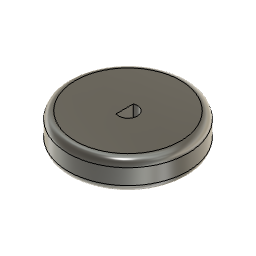
Full-Cat v5 (Autodesk Fusion 360 archive; units mm, degrees)
design "wheel v2"
Autodesk Fusion 360 part; units mm, degrees
sketch "Sketch1" plane through (0, 0, 0) normal (0, 0, 1) x (1, 0, 0)
  circle A0 centre (0, 0) radius 10
  dimension "d1" = 20
  constraint coincident A0.centre origin
  measures "d1" diameter of A0
extrude "Extrude1" add sketch "Sketch1" along normal blind 5
fillet "Fillet1" radius 1.2 2 edges at (-9.3233, -3.6162, 5) (-9.3233, -3.6162, 0)
sketch "Sketch2" plane through (0, 0, 5) normal (0, 0, 1) x (-1, 0, 0)
  circle A0 centre (0, 0) radius 8.8
  circle A1 centre (0, 0) radius 1.55
  line L0 (0.55, 1.4491) -> (2.3002, 1.4491)
  line L1 (2.3002, 1.4491) -> (2.3002, -1.4465)
  line L2 (2.3002, -1.4465) -> (0.55, -1.4465)
  line L3 (0.55, -1.4465) -> (0.55, 1.4491)
  dimension "d6" = 3.1
  dimension "d7" = 0.55
  constraint concentric A0 A1
  constraint horizontal L0
  constraint vertical L1
  constraint horizontal L2
  constraint vertical L3
  constraint coincident A1 L0.start
  measures "d6" diameter of A1
  measures "d7" distance of A0.centre L3
extrude "Extrude2" cut sketch "Sketch2" against normal blind 50 contours A1 L2 L3 picked at (-0.1284, 0.5)

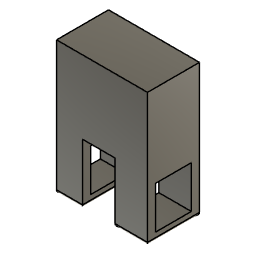
design "leg v11"
Autodesk Fusion 360 part; units mm, degrees
sketch "Sketch1" plane through (0, 0, 0) normal (0, 0, 1) x (1, 0, 0)
  line L0 (0, 0) -> (60, 0)
  line L1 (60, 0) -> (60, 20)
  line L2 (60, 20) -> (0, 20)
  line L3 (0, 20) -> (0, 0)
  dimension "d1" = 60
  dimension "d2" = 20
  constraint horizontal L0
  constraint vertical L1
  constraint horizontal L2
  constraint vertical L3
  constraint coincident L0.start L3.end
  measures "d1" distance of L0.start L0.end
  measures "d2" distance of L0.start L2.end
extrude "Extrude1" add sketch "Sketch1" along normal blind 40
sketch "Sketch2" plane through (0, 0, 0) normal (-1, 0, 0) x (0, -1, 0)
  line L0 (-20, 0) -> (0, 0)
  line L1 (0, 0) -> (0, 40)
  line L2 (0, 40) -> (-20, 40)
  line L3 (-20, 40) -> (-20, 0)
  line L4 (-15, 28) -> (-5, 28)
  line L5 (-5, 28) -> (-5, 16)
  line L6 (-5, 16) -> (-15, 16)
  line L7 (-15, 16) -> (-15, 28)
  dimension "d5" = 10
  dimension "d6" = 12
  dimension "d7" = 5
  constraint horizontal L4
  constraint vertical L5
  constraint horizontal L6
  constraint vertical L7
  measures "d5" distance of L4.start L4.end
  measures "d6" distance of L4.start L6.end
  measures "d7" distance of L3 L7
extrude "Extrude2" cut sketch "Sketch2" against normal blind 30 contours L4 L5 L6 L7
extrude "Extrude3" cut 1 faces at (20, 13.3333, 40) along direction (0, 0, -1) blind 2
extrude "Extrude4" cut 1 faces at (20, 13.3333, 0) along direction (0, 0, 1) blind 2
sketch "Sketch3" plane through (0, 20, 0) normal (0, 1, 0) x (-1, 0, 0)
  line L0 (-60, 2) -> (0, 2)
  line L1 (0, 2) -> (0, 38)
  line L2 (0, 38) -> (-60, 38)
  line L3 (-60, 38) -> (-60, 2)
  line L4 (-40, 33) -> (-20, 33)
  line L5 (-20, 33) -> (-20, -1)
  line L6 (-20, -1) -> (-40, -1)
  line L7 (-40, -1) -> (-40, 33)
  dimension "d14" = 20
  dimension "d15" = 34
  dimension "d16" = 20
  dimension "d17" = 5
  constraint horizontal L4
  constraint vertical L5
  constraint horizontal L6
  constraint vertical L7
  measures "d14" distance of L4.start L4.end
  measures "d15" distance of L4.start L6.end
  measures "d16" distance of L3 L7
  measures "d17" distance of L2 L4
extrude "Extrude5" cut 1 faces at (20, 13.3333, 2) along direction (0, 0, 1) blind 9
extrude "Extrude6" cut 1 faces at (20, 13.3333, 11) along direction (0, 0, 1) blind 1
extrude "Extrude7" cut sketch "Sketch3" against normal blind 20 contours L0 L4 L5 L7
extrude "Extrude8" cut sketch "Sketch2" against normal blind 80 contours L4 L5 L6 L7
extrude "Extrude9" cut 1 faces at (20, 13.3333, 38) along direction (0, 0, -1) blind 1
extrude "Extrude10" cut 1 faces at (60, 8.3333, 34) along direction (-1, 0, 0) blind 10
extrude "Extrude11" add 1 faces at (40, 1.6667, 24.3333) along direction (-1, 0, 0) blind 10
extrude "Extrude12" cut 1 faces at (50, 8.3333, 34) along direction (-1, 0, 0) blind 10
extrude "Extrude13" cut 1 faces at (6.6667, 20, 27.3333) along direction (0, -1, 0) blind 2
extrude "Extrude14" cut 1 faces at (6.6667, 0, 27.3333) along direction (0, 1, 0) blind 2
extrude "Extrude15" cut 1 faces at (36.6667, 12.6667, 12) along direction (0, 0, 1) blind 1
extrude "Extrude16" cut 1 faces at (13.3333, 7.3333, 12) along direction (0, 0, 1) blind 1
extrude "Extrude17" cut 1 faces at (36.6667, 12.6667, 13) along direction (0, 0, 1) blind 1
extrude "Extrude18" cut 1 faces at (13.3333, 7.3333, 13) along direction (0, 0, 1) blind 1
extrude "Extrude19" cut sketch "Sketch2" against normal blind 2
extrude "Extrude20" cut 1 faces at (14.6667, 7.3333, 37) along direction (0, 0, -1) blind 1
extrude "Extrude21" add 1 faces at (26.6667, 12.6667, 33) along direction (0, 0, -1) blind 1
extrude "Extrude22" cut 1 faces at (14.6667, 7.3333, 36) along direction (0, 0, -1) blind 1
fillet "Fillet1" radius 1 2 faces at (36.6667, 12.6667, 14) (14, 7.3333, 14)
sketch "Sketch4" plane through (2, 0, 0) normal (-1, 0, 0) x (0, -1, 0)
  line L0 (-5, 16) -> (-15, 16)
  line L1 (-15, 16) -> (-15, 28)
  line L2 (-15, 28) -> (-5, 28)
  line L3 (-5, 28) -> (-5, 16)
  line L4 (-18, 15) -> (-2, 15)
  line L5 (-2, 15) -> (-2, 35)
  line L6 (-2, 35) -> (-18, 35)
  line L7 (-18, 35) -> (-18, 15)
  line L8 (-15.5, 28.5) -> (-4.5, 28.5)
  line L9 (-4.5, 28.5) -> (-4.5, 15.5)
  line L10 (-4.5, 15.5) -> (-15.5, 15.5)
  line L11 (-15.5, 15.5) -> (-15.5, 28.5)
  dimension "d56" = 11
  dimension "d57" = 13
  dimension "d58" = 2.5
  dimension "d59" = 6.5
  constraint horizontal L8
  constraint vertical L9
  constraint horizontal L10
  constraint vertical L11
  measures "d56" distance of L8.start L8.end
  measures "d57" distance of L8.start L10.end
  measures "d58" distance of L7 L11
  measures "d59" distance of L6 L8
extrude "Extrude23" cut sketch "Sketch4" against normal blind 50 contours L8 L9 L10 L11
extrude "Extrude24" add 2 faces at (36.6667, 8.1667, 15.5) (14, 11.8333, 15.5) along direction (0, 0, 1) blind 1
extrude "Extrude25" cut 2 faces at (33.3333, 11.8333, 28.5) (14, 11.8333, 28.5) along direction (0, 0, 1) blind 1
extrude "Extrude26" cut 1 faces at (26.6667, 12.6667, 32) along direction (0, 0, 1) blind 0.5
extrude "Extrude27" add 1 faces at (14.6667, 7.3333, 35) along direction (0, 0, 1) blind 20
extrude "Extrude28" cut 1 faces at (2, 8.1667, 46.5) along direction (1, 0, 0) blind 10
extrude "Extrude29" cut 1 faces at (5.3333, 12.6667, 15) along direction (0, 0, -1) blind 15

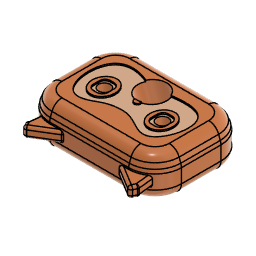
design "head v3"
Autodesk Fusion 360 part; units mm, degrees
sketch "Sketch1" plane through (0, 0, 0) normal (0, 0, 1) x (1, 0, 0)
  line L0 (10, 0) -> (40, 0)
  line L1 (50, 10) -> (50, 25)
  line L2 (40, 35) -> (10, 35)
  line L3 (0, 25) -> (0, 10)
  arc A0 (0, 10) -> (10, 0) centre (10, 10) ccw
  arc A1 (40, 0) -> (50, 10) centre (40, 10) ccw
  arc A2 (50, 25) -> (40, 35) centre (40, 25) ccw
  arc A3 (10, 35) -> (0, 25) centre (10, 25) ccw
  point P0 (50, 0)
  point P1 (0, 35)
  dimension "d1" = 50
  dimension "d2" = 35
  dimension "d3" = 10
  dimension "d4" = 10
  dimension "d5" = 10
  dimension "d6" = 10
  constraint horizontal L0
  constraint vertical L1
  constraint horizontal L2
  constraint vertical L3
  constraint coincident origin L0
  constraint coincident origin L3
  constraint tangent L0 A0
  constraint tangent L3 A0
  constraint coincident P0 L0
  constraint coincident P0 L1
  constraint tangent L0 A1
  constraint tangent L1 A1
  constraint tangent L1 A2
  constraint tangent L2 A2
  constraint coincident P1 L2
  constraint coincident P1 L3
  constraint tangent L2 A3
  constraint tangent L3 A3
  measures "d1" distance of origin P0
  measures "d2" distance of origin P1
  measures "d3" radius of A0
  measures "d4" radius of A1
  measures "d5" radius of A2
  measures "d6" radius of A3
extrude "Extrude1" add sketch "Sketch1" along normal blind 10 makes body 1
extrude "Extrude2" add 1 faces at (20, 23.3333, 10) along direction (0, 0, 1) blind 5 draft -20 on bodies 1 bodies 1
fillet "Fillet1" radius 4 16 faces at (9.2077, 34.0555, 12.5) (30, 34.3934, 11.6667) (49.0555, 25.7923, 12.5) (49.3934, 15, 11.6667) (49.0555, 9.2077, 12.5) (20, 0.6066, 11.6667) (9.2077, 0.9445, 12.5) (1.2132, 15, 13.3333) (0.2819, 27.3576, 6.6667) (0, 20, 3.3333) (8.1075, 0.1807, 6.6667) (20, 0, 3.3333) (40.4758, 0.0113, 6.6667) (50, 15, 3.3333) (40.4758, 34.9887, 6.6667) (30, 35, 3.3333) on bodies 1
sketch "Sketch2" plane through (0, 0, 15) normal (0, 0, 1) x (-1, 0, 0)
  arc A0 (-10, -30.3793) -> (-4.6207, -25) centre (-10, -25) ccw
  line L0 (-4.6207, -25) -> (-4.6207, -10)
  arc A1 (-4.6207, -10) -> (-10, -4.6207) centre (-10, -10) ccw
  line L1 (-10, -4.6207) -> (-40, -4.6207)
  arc A2 (-40, -4.6207) -> (-45.3793, -10) centre (-40, -10) ccw
  line L2 (-45.3793, -10) -> (-45.3793, -25)
  arc A3 (-45.3793, -25) -> (-40, -30.3793) centre (-40, -25) ccw
  line L3 (-40, -30.3793) -> (-10, -30.3793)
  spline S0 degree 5 poles (-30, -11) (-30.1783, -10.9228) (-30.547, -10.7574) (-31.1363, -10.4766) (-31.9947, -10.0363) (-33.1875, -9.3975) (-34.4939, -8.7332) (-35.9004, -8.1781) (-37.3826, -7.9333) (-38.9002, -8.1993) (-40.3935, -9.1277) (-41.777, -10.756) (-42.9392, -12.974) (-43.7599, -15.5782) (-44.125, -18.3111) (-43.9424, -20.9044) (-43.1572, -23.1215) (-41.7684, -24.7994) (-39.846, -25.8922) (-37.5109, -26.4441) (-34.9163, -26.5618) (-32.2287, -26.3888) (-29.6089, -26.0789) (-27.1947, -25.7719) (-25.0786, -25.5642) (-23.3123, -25.5105) (-22.1979, -25.6122) (-21.5328, -25.7732) (-21.165, -25.9181) (-21, -26) knots 0 0 0 0 0 0 0.04 0.08 0.12 0.16 0.2 0.24 0.28 0.32 0.36 0.4 0.44 0.48 0.52 0.56 0.6 0.64 0.68 0.72 0.76 0.8 0.84 0.88 0.92 0.96 1 1 1 1 1 1
  spline S1 degree 5 poles (-30, -11) (-29.7784, -11.1039) (-29.3296, -11.2982) (-28.6391, -11.549) (-27.6842, -11.8023) (-26.437, -11.984) (-25.1478, -12.0335) (-23.84, -11.9573) (-22.5543, -11.7675) (-21.3346, -11.4794) (-20.2112, -11.1086) (-19.1868, -10.6682) (-18.2159, -10.1651) (-17.224, -9.6104) (-16.1378, -9.036) (-14.9108, -8.5076) (-13.5535, -8.1426) (-12.1194, -8.0819) (-10.6872, -8.4572) (-9.346, -9.3624) (-8.176, -10.8165) (-7.2413, -12.7559) (-6.5937, -15.0609) (-6.2733, -17.5726) (-6.3103, -20.1129) (-6.7267, -22.5039) (-7.5371, -24.5856) (-8.75, -26.2385) (-10.3695, -27.3818) (-12.3961, -27.9646) (-14.8283, -27.9594) (-17.0966, -27.4759) (-18.9783, -26.8429) (-20.3128, -26.301) (-21, -26) knots 0 0 0 0 0 0 0.033333 0.066667 0.1 0.133333 0.166667 0.2 0.233333 0.266667 0.3 0.333333 0.366667 0.4 0.433333 0.466667 0.5 0.533333 0.566667 0.6 0.633333 0.666667 0.7 0.733333 0.766667 0.8 0.833333 0.866667 0.9 0.933333 0.966667 1 1 1 1 1 1
  point P0 (-34, -9)
  point P1 (-40, -9)
  point P2 (-43, -23)
  point P3 (-29, -26)
  point P4 (-25, -12)
  point P5 (-20, -11)
  point P6 (-16, -9)
  point P7 (-10, -9)
  point P8 (-7, -23)
extrude "Extrude3" cut sketch "Sketch2" against normal blind 0.5 contours S0 S1 bodies 1
sketch "Sketch3" plane through (0, 0, 14.5) normal (0, 0, 1) x (-1, 0, 0)
  spline S0 degree 5 poles (-21, -26) (-21.165, -25.9181) (-21.5328, -25.7732) (-22.1979, -25.6122) (-23.3123, -25.5105) (-25.0786, -25.5642) (-27.1947, -25.7719) (-29.6089, -26.0789) (-32.2287, -26.3888) (-34.9163, -26.5618) (-37.5109, -26.4441) (-39.846, -25.8922) (-41.7684, -24.7994) (-43.1572, -23.1215) (-43.9424, -20.9044) (-44.125, -18.3111) (-43.7599, -15.5782) (-42.9392, -12.974) (-41.777, -10.756) (-40.3935, -9.1277) (-38.9002, -8.1993) (-37.3826, -7.9333) (-35.9004, -8.1781) (-34.4939, -8.7332) (-33.1875, -9.3975) (-31.9947, -10.0363) (-31.1363, -10.4766) (-30.547, -10.7574) (-30.1783, -10.9228) (-30, -11) knots -1 -1 -1 -1 -1 -1 -0.96 -0.92 -0.88 -0.84 -0.8 -0.76 -0.72 -0.68 -0.64 -0.6 -0.56 -0.52 -0.48 -0.44 -0.4 -0.36 -0.32 -0.28 -0.24 -0.2 -0.16 -0.12 -0.08 -0.04 0 0 0 0 0 0
  spline S1 degree 5 poles (-30, -11) (-29.7784, -11.1039) (-29.3296, -11.2982) (-28.6391, -11.549) (-27.6842, -11.8023) (-26.437, -11.984) (-25.1478, -12.0335) (-23.84, -11.9573) (-22.5543, -11.7675) (-21.3346, -11.4794) (-20.2112, -11.1086) (-19.1868, -10.6682) (-18.2159, -10.1651) (-17.224, -9.6104) (-16.1378, -9.036) (-14.9108, -8.5076) (-13.5535, -8.1426) (-12.1194, -8.0819) (-10.6872, -8.4572) (-9.346, -9.3624) (-8.176, -10.8165) (-7.2413, -12.7559) (-6.5937, -15.0609) (-6.2733, -17.5726) (-6.3103, -20.1129) (-6.7267, -22.5039) (-7.5371, -24.5856) (-8.75, -26.2385) (-10.3695, -27.3818) (-12.3961, -27.9646) (-14.8283, -27.9594) (-17.0966, -27.4759) (-18.9783, -26.8429) (-20.3128, -26.301) (-21, -26) knots 0 0 0 0 0 0 0.033333 0.066667 0.1 0.133333 0.166667 0.2 0.233333 0.266667 0.3 0.333333 0.366667 0.4 0.433333 0.466667 0.5 0.533333 0.566667 0.6 0.633333 0.666667 0.7 0.733333 0.766667 0.8 0.833333 0.866667 0.9 0.933333 0.966667 1 1 1 1 1 1
  ellipse E0 centre (-37.25, -19.25) end of major axis (-37.25, -14.25) minor radius 4.35
  line L0 (-37.25, -24.25) -> (-37.25, -14.25) construction
  line L1 (-32.9, -19.25) -> (-41.6, -19.25) construction
  ellipse E1 centre (-14, -18) end of major axis (-14, -13) minor radius 4.3564
  line L2 (-14, -23) -> (-14, -13) construction
  line L3 (-9.6436, -18) -> (-18.3564, -18) construction
  line L4 (-38, -16) -> (-36.5, -16)
  line L5 (-34.5, -18) -> (-34.5, -20.5)
  line L6 (-36.5, -22.5) -> (-38, -22.5)
  line L7 (-40, -20.5) -> (-40, -18)
  arc A0 (-38, -16) -> (-40, -18) centre (-38, -18) ccw
  arc A1 (-34.5, -18) -> (-36.5, -16) centre (-36.5, -18) ccw
  arc A2 (-36.5, -22.5) -> (-34.5, -20.5) centre (-36.5, -20.5) ccw
  arc A3 (-40, -20.5) -> (-38, -22.5) centre (-38, -20.5) ccw
  point P0 (-40, -16)
  point P1 (-40, -22.5)
  dimension "d15" = 5.5
  dimension "d16" = 6.5
  dimension "d17" = 2
  dimension "d18" = 8.7
  dimension "d19" = 1.6
  dimension "d20" = 1.75
  constraint coincident E0 L0.start
  constraint coincident E0 L0.end
  constraint coincident E0 L1.start
  constraint coincident E0 L1.end
  constraint vertical L0
  constraint coincident E1 L2.start
  constraint coincident E1 L2.end
  constraint coincident E1 L3.start
  constraint coincident E1 L3.end
  constraint vertical L2
  constraint horizontal L4
  constraint vertical L5
  constraint horizontal L6
  constraint vertical L7
  constraint coincident P0 L4
  constraint coincident P0 L7
  constraint tangent L4 A0
  constraint tangent L7 A0
  constraint tangent L4 A1
  constraint tangent L5 A1
  constraint equal A0 A1
  constraint tangent L5 A2
  constraint tangent L6 A2
  constraint equal A0 A2
  constraint coincident P1 L6
  constraint coincident P1 L7
  constraint tangent L6 A3
  constraint tangent L7 A3
  constraint equal A0 A3
  measures "d16" distance of P0 P1
  measures "d17" radius of A0
  measures "d19" distance of L1.end L7
  measures "d20" distance of L0.end L4
extrude "Extrude4" add sketch "Sketch3" along normal blind 0.5 separate body contours E0 makes body 2
move_body "Move1" bodies 2 to x (1, 0, 0) y (0, 1, 0) z (0, 0, 1) at (0, -3, 0)
copy_body "CopyPasteBodies1" bodies 2 makes body 3
move_body "Move2" bodies 3 to x (1, 0, 0) y (0, 1, 0) z (0, 0, 1) at (-23, 0, 0)
move_body "Move3" bodies 2 to x (1, 0, 0) y (0, 1, 0) z (0, 0, 1) at (-1, 0, 0)
sketch "Sketch4" plane through (0, 0, 14.5) normal (0, 0, 1) x (-1, 0, 0)
  spline S0 degree 5 poles (-21, -26) (-21.165, -25.9181) (-21.5328, -25.7732) (-22.1979, -25.6122) (-23.3123, -25.5105) (-25.0786, -25.5642) (-27.1947, -25.7719) (-29.6089, -26.0789) (-32.2287, -26.3888) (-34.9163, -26.5618) (-37.5109, -26.4441) (-39.846, -25.8922) (-41.7684, -24.7994) (-43.1572, -23.1215) (-43.9424, -20.9044) (-44.125, -18.3111) (-43.7599, -15.5782) (-42.9392, -12.974) (-41.777, -10.756) (-40.3935, -9.1277) (-38.9002, -8.1993) (-37.3826, -7.9333) (-35.9004, -8.1781) (-34.4939, -8.7332) (-33.1875, -9.3975) (-31.9947, -10.0363) (-31.1363, -10.4766) (-30.547, -10.7574) (-30.1783, -10.9228) (-30, -11) knots -1 -1 -1 -1 -1 -1 -0.96 -0.92 -0.88 -0.84 -0.8 -0.76 -0.72 -0.68 -0.64 -0.6 -0.56 -0.52 -0.48 -0.44 -0.4 -0.36 -0.32 -0.28 -0.24 -0.2 -0.16 -0.12 -0.08 -0.04 0 0 0 0 0 0
  spline S1 degree 5 poles (-30, -11) (-29.7784, -11.1039) (-29.3296, -11.2982) (-28.6391, -11.549) (-27.6842, -11.8023) (-26.437, -11.984) (-25.1478, -12.0335) (-23.84, -11.9573) (-22.5543, -11.7675) (-21.3346, -11.4794) (-20.2112, -11.1086) (-19.1868, -10.6682) (-18.2159, -10.1651) (-17.224, -9.6104) (-16.1378, -9.036) (-14.9108, -8.5076) (-13.5535, -8.1426) (-12.1194, -8.0819) (-10.6872, -8.4572) (-9.346, -9.3624) (-8.176, -10.8165) (-7.2413, -12.7559) (-6.5937, -15.0609) (-6.2733, -17.5726) (-6.3103, -20.1129) (-6.7267, -22.5039) (-7.5371, -24.5856) (-8.75, -26.2385) (-10.3695, -27.3818) (-12.3961, -27.9646) (-14.8283, -27.9594) (-17.0966, -27.4759) (-18.9783, -26.8429) (-20.3128, -26.301) (-21, -26) knots 0 0 0 0 0 0 0.033333 0.066667 0.1 0.133333 0.166667 0.2 0.233333 0.266667 0.3 0.333333 0.366667 0.4 0.433333 0.466667 0.5 0.533333 0.566667 0.6 0.633333 0.666667 0.7 0.733333 0.766667 0.8 0.833333 0.866667 0.9 0.933333 0.966667 1 1 1 1 1 1
  circle A0 centre (-25, -20) radius 1.5
  spline S2 degree 5 poles (-25, -23.5) (-25.1849, -23.5) (-25.5547, -23.4789) (-26.1037, -23.384) (-26.8018, -23.1453) (-27.5648, -22.7428) (-28.1729, -22.3425) (-28.5917, -22.0497) (-28.8021, -21.9454) (-28.804, -22.0619) (-28.6205, -22.3581) (-28.2883, -22.7526) (-27.8491, -23.1531) (-27.3391, -23.4918) (-26.7839, -23.7424) (-26.2014, -23.9032) (-25.604, -23.9876) (-25, -24.0127) (-24.396, -23.9876) (-23.7986, -23.9032) (-23.2161, -23.7424) (-22.6609, -23.4918) (-22.1509, -23.1531) (-21.7117, -22.7526) (-21.3795, -22.3581) (-21.196, -22.0619) (-21.1979, -21.9454) (-21.4083, -22.0497) (-21.8271, -22.3425) (-22.4352, -22.7428) (-23.1982, -23.1453) (-23.8963, -23.384) (-24.4453, -23.4789) (-24.8151, -23.5) (-25, -23.5) knots 0 0 0 0 0 0 0.033333 0.066667 0.1 0.133333 0.166667 0.2 0.233333 0.266667 0.3 0.333333 0.366667 0.4 0.433333 0.466667 0.5 0.533333 0.566667 0.6 0.633333 0.666667 0.7 0.733333 0.766667 0.8 0.833333 0.866667 0.9 0.933333 0.966667 1 1 1 1 1 1
  point P0 (-28.75, -22)
  point P1 (-28, -23)
  point P2 (-25, -24)
  point P3 (-22, -23)
  point P4 (-21.25, -22)
  dimension "d23" = 3
  measures "d23" diameter of A0
extrude "Extrude5" add sketch "Sketch4" along normal blind 0.5 contours A0 | S2 bodies 1
sketch "Sketch5" plane through (0, 0, 0) normal (0, 0, 1) x (1, 0, 0)
  line L0 (15, -5) -> (23, -15)
  line L1 (23, -15) -> (25, -13)
  line L2 (25, -13) -> (27, -5)
  line L3 (27, -5) -> (15, -5)
  constraint horizontal L3
extrude "Extrude6" add sketch "Sketch5" along normal blind 2 separate body makes body 4
extrude "Extrude7" add 1 faces at (22.3333, -7.6667, 2) along direction (0, 0, 1) blind 2 on bodies 4 bodies 4
move_body "Move4" bodies 4 to x (1, 0, 0) y (0, 1, 0) z (0, 0, 1) at (18, 0, 4.75)
move_body "Move5" bodies 4 to x (1, 0, 0) y (0, 1, 0) z (0, 0, 1) at (1, 7, 0)
move_body "Move6" bodies 4 to x (0.939693, 0.34202, 0) y (-0.34202, 0.939693, 0) z (0, 0, 1) at (3.7692, -13.3411, 0)
fillet "Fillet2" radius 1 3 edges at (46.5701, -5.212, 8.75) (47.1678, -3.9303, 6.75) (40.6729, 2.2191, 4.75) 5 faces at (38.6806, -2.0532, 7.4167) (42.8378, 0.1693, 8.75) (46.3709, -5.6393, 6.0833) (42.8378, 0.1693, 4.75) (46.8822, -1.1965, 7.4167) on bodies 4
move_body "Move7" bodies 4 to x (1, 0, 0) y (0, 1, 0) z (0, 0, 1) at (0, 0.5, 0)
copy_body "CopyPasteBodies2" bodies 4 makes body 5
move_body "Move8" bodies 5 to x (-1, 0, 0) y (0, 1, 0) z (0, 0, -1) at (51.6637, 0, 13.5)
combine "Combine1" operation add target body 1 tool bodies 5 4
scale "Scale1" factor 1.2 about (17, 17.5, 14.5) bodies 2 1 3
extrude "Extrude8" add 1 faces at (24.7964, 24.5851, 15.1) along direction (0, 0, -1) blind 0.5 on bodies 1 bodies 1
extrude "Extrude9" cut 2 faces at (23.2881, 23.8355, 15.1) (26.9741, 20.4484, 15.1) along direction (0, 0, -1) blind 0.5 on bodies 1 bodies 1
extrude "Extrude10" cut 2 faces at (26.9741, 20.4484, 14.6) (23.2881, 23.8355, 14.6) along direction (0, 0, -1) blind 0.1 on bodies 1 bodies 1
sketch "Sketch7" plane through (0, 0, 0) normal (0, 0, 1) x (1, 0, 0)
cylinder "CylinderPrimitive1" add diameter 13 height 50 placed x (1, 0, 0) y (0, 1, 0) z (0, 0, 1) at (0, 0, 0) separate body makes body 6
move_body "Move9" bodies 6 to x (1, 0, 0) y (0, 1, 0) z (0, 0, 1) at (26.6, 26, -19)
sketch "Sketch9" plane through (0, 0, 14.5) normal (0, 0, 1) x (-1, 0, 0)
  spline S0 degree 5 poles (-21.8, -27.7) (-21.998, -27.6018) (-22.4393, -27.4279) (-23.2375, -27.2346) (-24.5747, -27.1127) (-26.6943, -27.177) (-29.2336, -27.4263) (-32.1306, -27.7946) (-35.2744, -28.1666) (-38.4995, -28.3742) (-41.6131, -28.2329) (-44.4152, -27.5707) (-46.7221, -26.2593) (-48.3886, -24.2458) (-49.3309, -21.5853) (-49.55, -18.4733) (-49.1118, -15.1939) (-48.127, -12.0688) (-46.7324, -9.4072) (-45.0722, -7.4532) (-43.2802, -6.3391) (-41.4591, -6.0199) (-39.6805, -6.3137) (-37.9927, -6.9798) (-36.425, -7.777) (-34.9937, -8.5435) (-33.9636, -9.072) (-33.2564, -9.4089) (-32.814, -9.6074) (-32.6, -9.7) knots -1 -1 -1 -1 -1 -1 -0.96 -0.92 -0.88 -0.84 -0.8 -0.76 -0.72 -0.68 -0.64 -0.6 -0.56 -0.52 -0.48 -0.44 -0.4 -0.36 -0.32 -0.28 -0.24 -0.2 -0.16 -0.12 -0.08 -0.04 0 0 0 0 0 0
  spline S1 degree 5 poles (-32.6, -9.7) (-32.3341, -9.8247) (-31.7955, -10.0578) (-30.9669, -10.3588) (-29.8211, -10.6628) (-28.3244, -10.8809) (-26.7773, -10.9402) (-25.208, -10.8488) (-23.6651, -10.621) (-22.2015, -10.2753) (-20.8534, -9.8303) (-19.6242, -9.3019) (-18.4591, -8.6981) (-17.2688, -8.0325) (-15.9654, -7.3432) (-14.493, -6.7092) (-12.8642, -6.2711) (-11.1433, -6.1983) (-9.4247, -6.6486) (-7.8152, -7.7349) (-6.4112, -9.4798) (-5.2895, -11.8071) (-4.5124, -14.5731) (-4.1279, -17.5871) (-4.1724, -20.6355) (-4.6721, -23.5047) (-5.6445, -26.0027) (-7.1001, -27.9862) (-9.0434, -29.3581) (-11.4753, -30.0575) (-14.394, -30.0513) (-17.116, -29.4711) (-19.3739, -28.7115) (-20.9753, -28.0611) (-21.8, -27.7) knots 0 0 0 0 0 0 0.033333 0.066667 0.1 0.133333 0.166667 0.2 0.233333 0.266667 0.3 0.333333 0.366667 0.4 0.433333 0.466667 0.5 0.533333 0.566667 0.6 0.633333 0.666667 0.7 0.733333 0.766667 0.8 0.833333 0.866667 0.9 0.933333 0.966667 1 1 1 1 1 1
  circle A0 centre (-27, -18) radius 1.4142
extrude "Extrude11" add sketch "Sketch9" along normal blind 0.5 contours A0 bodies 1
move_face "MoveFace1" to x (1, 0, 0) y (0, 0.965926, 0.258819) z (0, -0.258819, 0.965926) at (0, 3.2712, -7.7251) 1 faces at (33.0677, 25.3528, 14.3333) on bodies 6
move_body "Move10" bodies 6 to x (1, 0, 0) y (0, 1, 0) z (0, 0, 1) at (0, 1, 0)
combine "Combine2" operation cut target body 1 tool bodies 6
sketch "Sketch10" plane through (0, 0, 14.5) normal (0, 0, 1) x (-1, 0, 0)
  ellipse E0 centre (-26.6, -25.2331) end of major axis (-26.6, -31.9624) minor radius 6.5 (-20.7408, -28.1465) -> (-25.7048, -18.568) ccw
  spline S0 degree 5 poles (-32.6, -9.7) (-32.3341, -9.8247) (-31.7955, -10.0578) (-30.9669, -10.3588) (-29.8211, -10.6628) (-28.3244, -10.8809) (-26.7773, -10.9402) (-25.208, -10.8488) (-23.6651, -10.621) (-22.2015, -10.2753) (-20.8534, -9.8303) (-19.6242, -9.3019) (-18.4591, -8.6981) (-17.2688, -8.0325) (-15.9654, -7.3432) (-14.493, -6.7092) (-12.8642, -6.2711) (-11.1433, -6.1983) (-9.4247, -6.6486) (-7.8152, -7.7349) (-6.4112, -9.4798) (-5.2895, -11.8071) (-4.5124, -14.5731) (-4.1279, -17.5871) (-4.1724, -20.6355) (-4.6721, -23.5047) (-5.6445, -26.0027) (-7.1001, -27.9862) (-9.0434, -29.3581) (-11.4753, -30.0575) (-14.2417, -30.0516) (-16.7626, -29.5443) (-18.7899, -28.9022) (-20.1497, -28.3857) (-20.7408, -28.1465) knots 0 0 0 0 0 0 0.033333 0.066667 0.1 0.133333 0.166667 0.2 0.233333 0.266667 0.3 0.333333 0.366667 0.4 0.433333 0.466667 0.5 0.533333 0.566667 0.6 0.633333 0.666667 0.7 0.733333 0.766667 0.8 0.833333 0.866667 0.9 0.933333 0.966667 0.991305 0.991305 0.991305 0.991305 0.991305 0.991305
  spline S1 degree 5 poles (-32.5915, -27.8424) (-33.119, -27.9042) (-34.272, -28.0354) (-36.0898, -28.2188) (-38.5818, -28.3705) (-41.6131, -28.2329) (-44.4152, -27.5707) (-46.7221, -26.2593) (-48.3886, -24.2458) (-49.3309, -21.5853) (-49.55, -18.4733) (-49.1118, -15.1939) (-48.127, -12.0688) (-46.7324, -9.4072) (-45.0722, -7.4532) (-43.2802, -6.3391) (-41.4591, -6.0199) (-39.6805, -6.3137) (-37.9927, -6.9798) (-36.425, -7.777) (-34.9937, -8.5435) (-33.9636, -9.072) (-33.2564, -9.4089) (-32.814, -9.6074) (-32.6, -9.7) knots -0.794714 -0.794714 -0.794714 -0.794714 -0.794714 -0.794714 -0.76 -0.72 -0.68 -0.64 -0.6 -0.56 -0.52 -0.48 -0.44 -0.4 -0.36 -0.32 -0.28 -0.24 -0.2 -0.16 -0.12 -0.08 -0.04 0 0 0 0 0 0
  ellipse E1 centre (-26.6, -25.2331) end of major axis (-26.6, -31.9624) minor radius 6.5 (-28.2195, -18.7161) -> (-32.5915, -27.8424) ccw
  arc A0 (-25.7048, -18.568) -> (-28.2195, -18.7161) centre (-27, -18) ccw
  circle A1 centre (-40.162, -16.2865) radius 2.7
  dimension "d45" = 5.4
  measures "d45" diameter of A1
extrude "Extrude12" cut sketch "Sketch10" against normal blind 20 contours A1 bodies 1
sketch "Sketch11" plane through (0, 0, 14.5) normal (0, 0, 1) x (-1, 0, 0)
  circle A0 centre (-40.162, -16.2865) radius 2.7
  ellipse E0 centre (-26.6, -25.2331) end of major axis (-26.6, -31.9624) minor radius 6.5 (-20.7408, -28.1465) -> (-25.7048, -18.568) ccw
  spline S0 degree 5 poles (-32.6, -9.7) (-32.3341, -9.8247) (-31.7955, -10.0578) (-30.9669, -10.3588) (-29.8211, -10.6628) (-28.3244, -10.8809) (-26.7773, -10.9402) (-25.208, -10.8488) (-23.6651, -10.621) (-22.2015, -10.2753) (-20.8534, -9.8303) (-19.6242, -9.3019) (-18.4591, -8.6981) (-17.2688, -8.0325) (-15.9654, -7.3432) (-14.493, -6.7092) (-12.8642, -6.2711) (-11.1433, -6.1983) (-9.4247, -6.6486) (-7.8152, -7.7349) (-6.4112, -9.4798) (-5.2895, -11.8071) (-4.5124, -14.5731) (-4.1279, -17.5871) (-4.1724, -20.6355) (-4.6721, -23.5047) (-5.6445, -26.0027) (-7.1001, -27.9862) (-9.0434, -29.3581) (-11.4753, -30.0575) (-14.2417, -30.0516) (-16.7626, -29.5443) (-18.7899, -28.9022) (-20.1497, -28.3857) (-20.7408, -28.1465) knots 0 0 0 0 0 0 0.033333 0.066667 0.1 0.133333 0.166667 0.2 0.233333 0.266667 0.3 0.333333 0.366667 0.4 0.433333 0.466667 0.5 0.533333 0.566667 0.6 0.633333 0.666667 0.7 0.733333 0.766667 0.8 0.833333 0.866667 0.9 0.933333 0.966667 0.991305 0.991305 0.991305 0.991305 0.991305 0.991305
  spline S1 degree 5 poles (-32.5915, -27.8424) (-33.119, -27.9042) (-34.272, -28.0354) (-36.0898, -28.2188) (-38.5818, -28.3705) (-41.6131, -28.2329) (-44.4152, -27.5707) (-46.7221, -26.2593) (-48.3886, -24.2458) (-49.3309, -21.5853) (-49.55, -18.4733) (-49.1118, -15.1939) (-48.127, -12.0688) (-46.7324, -9.4072) (-45.0722, -7.4532) (-43.2802, -6.3391) (-41.4591, -6.0199) (-39.6805, -6.3137) (-37.9927, -6.9798) (-36.425, -7.777) (-34.9937, -8.5435) (-33.9636, -9.072) (-33.2564, -9.4089) (-32.814, -9.6074) (-32.6, -9.7) knots -0.794714 -0.794714 -0.794714 -0.794714 -0.794714 -0.794714 -0.76 -0.72 -0.68 -0.64 -0.6 -0.56 -0.52 -0.48 -0.44 -0.4 -0.36 -0.32 -0.28 -0.24 -0.2 -0.16 -0.12 -0.08 -0.04 0 0 0 0 0 0
  ellipse E1 centre (-26.6, -25.2331) end of major axis (-26.6, -31.9624) minor radius 6.5 (-28.2195, -18.7161) -> (-32.5915, -27.8424) ccw
  arc A1 (-25.7048, -18.568) -> (-28.2195, -18.7161) centre (-27, -18) ccw
  circle A2 centre (-13.7331, -16.2693) radius 2.7
  dimension "d48" = 5.4
  measures "d48" diameter of A2
extrude "Extrude13" cut sketch "Sketch11" against normal blind 20 contours A2 bodies 1
combine "Combine3" operation add target body 1 tool bodies 2 3
scale "Scale2" factor 1.5 about (51.0552, 8.5, 15.1) bodies 1

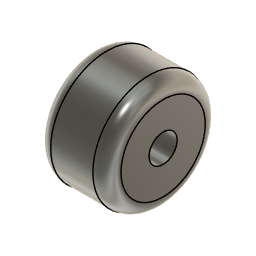
design "FlyWheel-Bot"
Autodesk Fusion 360 part; units mm, degrees
sketch "Sketch1" plane through (0, 0, 0) normal (1, 0, 0) x (0, 1, 0)
  circle A0 centre (0, 0) radius 1
  circle A1 centre (0, 0) radius 4
  dimension "d1" = 2
  dimension "d2" = 8
  constraint coincident A0.centre A1.centre
  measures "d1" diameter of A0
  measures "d2" diameter of A1
extrude "Extrude1" add sketch "Sketch1" along normal blind 5
fillet "Fillet1" radius 1 1 edges at (0, -3.7293, -1.4465)
fillet "Fillet2" radius 1 1 edges at (5, -3.7293, -1.4465)
